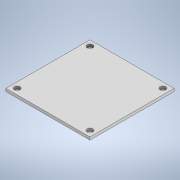
# Autodesk Inventor part: down side
Saved by Autodesk Inventor 2021 (Build 250183000, 183)
## iProperties
Created: 2021-07-01
Part Number: down side
Material: Generic
Document SubType Name: Modeling
Designer: almas
Density: 1 g/cm^3
Appearance: Default
Author: almas
Autodesk Inventor part; units mm, degrees
ref_plane "YZ Plane" through (0, 0, 0) normal (1, 0, 0) x (0, 1, 0)
ref_plane "XZ Plane" through (0, 0, 0) normal (0, 1, 0) x (-1, 0, 0)
ref_plane "XY Plane" through (0, 0, 0) normal (0, 0, 1) x (1, 0, 0)
sketch "Sketch1" plane through (0, 0, 0) normal (0, 1, 0) x (-1, 0, 0)
  line L0 (0, 0) -> (381, 0)
  line L1 (381, 0) -> (381, -381)
  line L2 (381, -381) -> (0, -381)
  line L3 (0, -381) -> (0, 0)
  constraints: 8 end point, 2 parallel, 1 horizontal, 1 perpendicular
extrude "Extrusion1" add sketch "Sketch1" along normal blind 12.7
sketch "Sketch2" plane through (0, 12.7, 0) normal (0, 1, 0) x (1, 0, 0)
  circle A0 centre (-25.4, 25.4) radius 12.7
  line L0 (0, 0) -> (0, 381) projected
  line L1 (-381, 0) -> (0, 0) projected
  constraints: 1 centre point
extrude "Extrusion2" cut sketch "Sketch2" against normal blind 12.7
sketch "Sketch3" plane through (0, 12.7, 0) normal (0, 1, 0) x (1, 0, 0)
  circle A0 centre (-25.4, 355.6) radius 12.7
  line L0 (0, 381) -> (-381, 381) projected
  line L1 (0, 0) -> (0, 381) projected
  constraints: 1 centre point
extrude "Extrusion3" cut sketch "Sketch3" against normal blind 12.7
sketch "Sketch4" plane through (0, 12.7, 0) normal (0, 1, 0) x (1, 0, 0)
  circle A0 centre (-355.6, 25.4) radius 12.7
  line L0 (-381, 381) -> (-381, 0) projected
  line L1 (-381, 0) -> (0, 0) projected
  constraints: 1 centre point
extrude "Extrusion4" cut sketch "Sketch4" against normal blind 12.7
sketch "Sketch5" plane through (0, 12.7, 0) normal (0, 1, 0) x (1, 0, 0)
  circle A0 centre (-355.6, 355.6) radius 12.7
  line L0 (0, 381) -> (-381, 381) projected
  line L1 (-381, 381) -> (-381, 0) projected
  point P0 (0, 0)
  constraints: 1 centre point
extrude "Extrusion5" cut sketch "Sketch5" against normal blind 12.7
body "Solid1"
